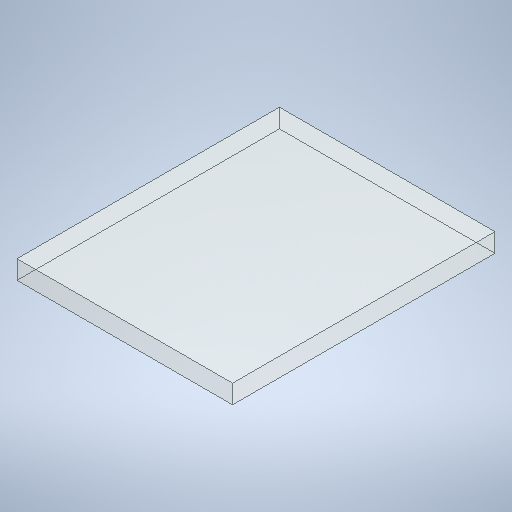
# Autodesk Inventor part: Cover
Saved by Autodesk Inventor 2025.2 (Build 292293000, 293)
## iProperties
Created: 2025-06-17
Part Number: Cover
Material: Glass
Document SubType Name: Modeling
Designer: user
Density: 2.18 g/cm^3
Appearance: Clear
Author: user
Autodesk Inventor part; units mm, degrees
ref_plane "YZ Plane" through (0, 0, 0) normal (1, 0, 0) x (0, 1, 0)
ref_plane "XZ Plane" through (0, 0, 0) normal (0, 1, 0) x (-1, 0, 0)
ref_plane "XY Plane" through (0, 0, 0) normal (0, 0, 1) x (1, 0, 0)
sketch "Sketch1" plane through (0, 0, 0) normal (0, 0, 1) x (1, 0, 0)
  line L0 (-11.5, 1) -> (11.5, 1)
  line L1 (11.5, 1) -> (11.5, -1)
  line L2 (11.5, -1) -> (-11.5, -1)
  line L3 (-11.5, -1) -> (-11.5, 1)
  point P0 (0, 0)
  dimension "d0" = 23
  dimension "d1" = 2
  dimension "d2" = 1
  dimension "d3" = 11.5
  constraints: 8 end point, 2 parallel, 1 horizontal, 1 perpendicular
  measures "d0" distance of L1.end L2.end
  measures "d1" distance of L0.end L1.end
  measures "d2" distance from line of point (0, 0) L0
  measures "d3" distance from line of point (0, 0) L3
extrude "Extrusion1" add sketch "Sketch1" along normal blind 28
equation "\"d2\" = 0.5 * d1"
equation "\"d3\" = 0.5 * d0"
body "Solid1"
